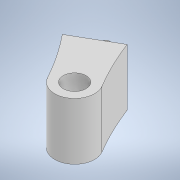
# Autodesk Inventor part: screw in stablity
Saved by Autodesk Inventor 2020 (Build 240168000, 168)
## iProperties
Created: 2019-07-11
Part Number: screw in stablity
Material: Generic
Document SubType Name: Modeling
Designer: ColinP
Density: 1 g/cm^3
Appearance: Default
Author: ColinP
Autodesk Inventor part; units mm, degrees
ref_plane "YZ Plane" through (0, 0, 0) normal (1, 0, 0) x (0, 1, 0)
ref_plane "XZ Plane" through (0, 0, 0) normal (0, 1, 0) x (-1, 0, 0)
ref_plane "XY Plane" through (0, 0, 0) normal (0, 0, 1) x (1, 0, 0)
sketch "Sketch1" plane through (0, 0, 0) normal (0, 1, 0) x (-1, 0, 0)
  line L0 (0, 0) -> (28.575, 0)
  line L1 (28.575, 0) -> (0, 0)
  line L2 (0, 0) -> (-14.2875, -24.7467)
  line L3 (0, 0) -> (28.575, 0) construction
  line L4 (0, 0) -> (-14.2875, 24.7467)
  line L5 (0, 0) -> (28.575, 0) construction
  circle A0 centre (28.575, 0) radius 2.54
  circle A1 centre (-14.2875, -24.7467) radius 2.54
  circle A2 centre (-14.2875, 24.7467) radius 2.54
  circle A3 centre (0, 0) radius 3.175
  dimension "d0" = 28.575
  dimension "d1" = 28.575
  dimension "d2" = 120
  dimension "d3" = 28.575
  dimension "d4" = 120
  dimension "d5" = 5.08
  dimension "d6" = 5.08
  dimension "d7" = 5.08
  dimension "d9" = 6.35
  constraints: 12 end point, 4 centre point, 4 coincident, 3 horizontal, 2 equal length, 1 collinear
  measures "d0" distance of L0.start L0.end
  measures "d1" distance of L0.start L2.end
  measures "d2" angle of L2 L3
  measures "d3" distance of L0.start L4.end
  measures "d4" angle of L5 L4
  measures "d5" diameter of A0
  measures "d6" diameter of A1
  measures "d7" diameter of A2
  measures "d9" diameter of A3
sketch "Sketch2" plane through (0, 0, 0) normal (0, 1, 0) x (-1, 0, 0)
  circle A0 centre (28.575, 0) radius 2.54 projected
  circle A1 centre (-14.2875, -24.7467) radius 2.54 projected
  circle A2 centre (-14.2875, 24.7467) radius 2.54 projected
  circle A3 centre (28.575, 0) radius 4.445
  circle A4 centre (-14.2875, -24.7467) radius 4.445
  circle A5 centre (-14.2875, 24.7467) radius 4.445
  circle A6 centre (0, 0) radius 6.35
  circle A7 centre (0, 0) radius 9.525
  line L0 (28.575, 4.445) -> (28.575, -4.445)
  line L1 (-14.2875, 24.7467) -> (0, 0)
  line L2 (0, 0) -> (-14.2875, 24.7467)
  line L3 (-14.2875, 24.7467) -> (-10.438, 26.9692)
  line L4 (-14.2875, 24.7467) -> (-18.137, 22.5242)
  line L5 (0, 0) -> (-14.2875, -24.7467)
  line L6 (-10.438, -26.9692) -> (-14.2875, -24.7467)
  line L7 (-18.137, -22.5242) -> (-14.2875, -24.7467)
  arc A8 (4.7625, 8.2489) -> (28.575, 4.445) centre (26.9969, 71.0017) ccw
  arc A9 (28.575, -4.445) -> (4.7625, -8.2489) centre (26.881, -70.2762) ccw
  arc A10 (4.7625, -8.2489) -> (-10.438, -26.9692) centre (47.4204, -58.4177) ccw
  arc A11 (-18.137, -22.5242) -> (-9.525, 0) centre (-74.3014, 11.8584) ccw
  arc A12 (-9.525, 0) -> (-18.137, 22.5242) centre (-78.365, -13.4121) ccw
  arc A13 (-10.438, 26.9692) -> (4.7625, 8.2489) centre (47.4204, 58.4177) ccw
  arc A14 (-3.702, 16.9073) -> (16.4951, 5.2598) centre (24.8224, 43.0343) ccw
  arc A15 (16.4931, -5.2477) -> (-3.702, -16.9073) centre (24.8816, -43.0963) ccw
  line L8 (-9.525, 0) -> (-10.9982, 0)
  arc A16 (-12.7912, -11.6596) -> (-12.8557, 11.635) centre (-49.0728, -0.1126) ccw
  dimension "d10" = 8.89
  dimension "d11" = 8.89
  dimension "d12" = 8.89
  dimension "d13" = 12.7
  dimension "d14" = 19.05
  dimension "d15" = 1.4732
  constraints: 31 point on circle, 18 end point, 14 centre point, 5 coincident, 3 perpendicular, 1 collinear, 1 horizontal, 1 line through centre, 1 point on line, 1 vertical
  measures "d10" diameter of A3
  measures "d11" diameter of A4
  measures "d12" diameter of A5
  measures "d13" diameter of A6
  measures "d14" diameter of A7
  measures "d15" distance of L8.start L8.end
extrude "Extrusion1" add sketch "Sketch2" along normal blind 12.7 contours A0 L0 A3 | A0 L0 A9 A7 A8 | L6 A1 L5 A4 | A11 A7 L5 A4 | L4 A2 L1 A5 | A13 A7 L1 A5 | A8 A13 A14 | A15 A10 A9 | A7 L5 A6 L1 | A4 L7 A1 L6 | A10 A4 L5 A7 | L1 A6 L5 A7 | A5 L3 A2 L4 | A7 A12 A5 L1 | A5 L1 A2 L3 | L8 A16 A12 | A11 A16 L8 | L1 L5 A6 | A6 L5 L1 | L5 A1 L7 A4
hole "Hole1" at (0, 0, 0) direction (0, 1, 0) diameter 6.35 end through all
sketch "Sketch3" plane through (0, 12.7, 0) normal (0, 1, 0) x (1, 0, 0)
  circle A0 centre (0, 0) radius 3.175 projected
  constraints: 1 coincident
hole "Hole2" at (0, 12.7, 0) direction (0, -1, 0) diameter 6.604 end through all
sketch "Sketch4" plane through (0, 12.7, 0) normal (0, 1, 0) x (1, 0, 0)
  circle A0 centre (-10.3993, 5.2212) radius 3.175 projected
  circle A1 centre (-10.8149, -4.2948) radius 3.175 projected
  point P0 (0, 0)
hole "Hole3" at (-10.3993, 12.7, -5.2212) at (-10.8149, 12.7, 4.2948) direction (0, -1, 0) diameter 6.35 depth 162.56
sketch "Sketch5" plane through (0, 12.7, 0) normal (0, 1, 0) x (1, 0, 0)
  arc A0 (-16.4951, -5.2598) -> (-28.575, -4.445) centre (-26.9969, -71.0017) ccw projected
  arc A1 (-28.575, 4.445) -> (-16.4931, 5.2477) centre (-26.881, 70.2762) ccw projected
  line L0 (-16.4951, -5.2598) -> (-16.4931, 5.2477)
  arc A2 (10.438, -26.9692) -> (3.702, -16.9073) centre (-47.4204, -58.4177) ccw projected
  arc A3 (12.8557, -11.635) -> (18.137, -22.5242) centre (78.365, 13.4121) ccw projected
  line L1 (3.702, -16.9073) -> (12.8557, -11.635)
  arc A4 (18.137, 22.5242) -> (12.7912, 11.6596) centre (74.3014, -11.8584) ccw projected
  arc A5 (3.702, 16.9073) -> (10.438, 26.9692) centre (-47.4204, 58.4177) ccw projected
  line L2 (12.7912, 11.6596) -> (3.702, 16.9073)
  arc A6 (18.137, 22.5242) -> (10.438, 26.9692) centre (14.2875, 24.7467) ccw projected
  arc A7 (-28.575, 4.445) -> (-28.575, -4.445) centre (-28.575, 0) ccw projected
  point P0 (0, 0)
  constraints: 6 end point
sketch "Sketch6" plane through (0, 12.7, 0) normal (0, 1, 0) x (1, 0, 0)
  arc A0 (-13.4646, 6.0485) -> (-8.668, 7.8826) centre (-10.3993, 5.2212) ccw projected
  line L0 (-10.3993, 5.2212) -> (-7.2243, 5.2212)
  line L1 (-10.3993, 5.2212) -> (-13.5743, 5.2212)
  line L2 (-13.5743, 5.2212) -> (-13.5743, 8.7596)
  line L3 (-13.5743, 8.7596) -> (-7.2855, 8.8652)
  line L4 (-7.2855, 8.8652) -> (-7.2243, 5.2212)
  arc A1 (-9.9167, -7.3401) -> (-13.4529, -6.0614) centre (-10.8149, -4.2948) ccw projected
  line L5 (-10.8149, -4.2948) -> (-13.9899, -4.2948)
  line L6 (-13.9899, -4.2948) -> (-13.9899, -9.3241)
  line L7 (-10.8149, -4.2948) -> (-7.6399, -4.2948)
  line L8 (-7.6399, -4.2948) -> (-7.6399, -9.0772)
  line L9 (-7.6399, -9.0772) -> (-13.9899, -9.3241)
  point P0 (0, 0)
  constraints: 20 end point, 4 point on circle, 3 horizontal, 3 vertical, 2 tangent, 1 perpendicular, 1 point on line
extrude "Extrusion2" cut sketch "Sketch6" against normal blind 25.4 contours L2 L3 L4 L0 L1 | L8 L9 L6 L5 L7
sketch "Sketch7" plane through (0, 12.7, 0) normal (0, 1, 0) x (1, 0, 0)
  arc A0 (12.7912, 11.6596) -> (12.8557, -11.635) centre (49.0728, 0.1126) ccw projected
  arc A1 (12.7912, 11.6596) -> (12.8557, -11.635) centre (49.0728, 0.1126) ccw
  arc A2 (-7.2803, 8.5554) -> (3.702, 16.9073) centre (-24.8816, 43.0963) ccw projected
  arc A3 (-16.4931, 5.2477) -> (3.702, 16.9073) centre (-24.8816, 43.0963) ccw
  arc A4 (-13.9899, -5.9006) -> (-16.4951, -5.2598) centre (-24.8224, -43.0343) ccw projected
  arc A5 (3.702, -16.9073) -> (-16.4951, -5.2598) centre (-24.8224, -43.0343) ccw
  arc A6 (-28.575, 4.445) -> (-16.4931, 5.2477) centre (-26.881, 70.2762) ccw projected
  line L0 (-16.4931, 5.2477) -> (-16.4951, -5.2598)
  line L1 (3.702, -16.9073) -> (12.8557, -11.635)
  line L2 (3.702, 16.9073) -> (12.7912, 11.6596)
  point P0 (0, 0)
  point P1 (-7.2803, 8.5554)
  point P2 (-13.9899, -5.9006)
  constraints: 6 end point, 6 point on circle, 3 centre point
extrude "Extrusion3" cut sketch "Sketch7" against normal blind 25.4
extrude "Extrusion4" cut sketch "Sketch5" against normal blind 25.4
sketch "Sketch9" plane through (3.702, 0, 16.9073) normal (-0.4991072, 0, -0.8665403) x (-0.8665403, 0, 0.4991072)
  line L0 (0, 0) -> (0, 12.7) projected
  line L1 (0, 6.35) -> (-10.5635, 6.35)
  line L2 (-10.5635, 0) -> (-10.5635, 12.7) projected
  line L3 (-7.8001, 12.7) -> (-2.7201, 12.7) projected
  line L4 (-5.2601, 12.7) -> (-5.2307, 0)
  circle A0 centre (-5.2454, 6.35) radius 1.0065
  dimension "d45" = 2.013
  constraints: 4 end point, 4 midpoint, 1 centre point, 1 coincident
  measures "d45" diameter of A0
extrude "Extrusion5" add sketch "Sketch9" along normal blind 7.5946
thread "Thread1" size "M2.5x0.45" class "6g" standard "ISO Metric profile" full length
body "Solid1"
